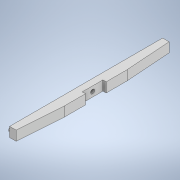
# Autodesk Inventor part: atx_mount
Saved by Autodesk Inventor 2022 (Build 260153000, 153)
## iProperties
Created: 2021-12-15
Part Number: atx_mount
Material: Generisch
Document SubType Name: Modeling
Designer: Niclas
Density: 1 g/cm^3
Appearance: Vorgabe
Author: Niclas
Autodesk Inventor part; units mm, degrees
ref_plane "YZ Plane" through (0, 0, 0) normal (1, 0, 0) x (0, 1, 0)
ref_plane "XZ Plane" through (0, 0, 0) normal (0, 1, 0) x (-1, 0, 0)
ref_plane "XY Plane" through (0, 0, 0) normal (0, 0, 1) x (1, 0, 0)
sketch "Skizze3" plane through (0, 0, 0) normal (0, 1, 0) x (-1, 0, 0)
  line L0 (15, 237) -> (0, 237)
  line L1 (0, 237) -> (0, 0)
  line L2 (0, 0) -> (15, 0)
  line L3 (15, 0) -> (15, 237)
  line L4 (5, 134.5) -> (0, 134.5)
  line L5 (0, 134.5) -> (0, 102.5)
  line L6 (0, 102.5) -> (5, 102.5)
  line L7 (5, 102.5) -> (5, 134.5)
  point P0 (0, 134.5)
  dimension "d17" = 237
  dimension "d18" = 15
  dimension "d19" = 5
  dimension "d20" = 32
  dimension "d69" = 102.5
  constraints: 16 end point, 4 parallel, 2 horizontal, 2 perpendicular, 1 coincident, 1 point on line
  measures "d17" distance of L2.end L0.start
  measures "d18" distance of L1.end L2.end
  measures "d19" distance of L5.end L6.end
  measures "d20" distance between parallel lines of L6 L4
  measures "d69" distance between parallel lines of L2 L6
extrude "Extrusion4" add sketch "Skizze3" along normal blind 15 contours L3 L2 L1 L6 L7 L4 L0
sketch "Skizze6" plane through (0, 0, 0) normal (0, -1, 0) x (1, 0, 0)
  line L0 (0, 70) -> (-5, 0)
  line L1 (0, 0) -> (-15, 0) projected
  line L2 (0, 102.5) -> (0, 0) projected
  line L3 (-5, 237) -> (0, 167)
  line L4 (-15, 237) -> (0, 237) projected
  line L5 (0, 237) -> (0, 134.5) projected
  point P0 (0, 167)
  dimension "d48" = 0
  dimension "d49" = 10
  dimension "d50" = 0
  dimension "d51" = 70
  dimension "d52" = 0
  dimension "d53" = 10
  dimension "d54" = 70
  dimension "d55" = 0
  constraints: 4 end point
  measures "d48" distance from line of L1 L0.end
  measures "d49" distance of L1.end L0.end
  measures "d50" distance from line of L2 L0.start
  measures "d51" distance of L0.start L1.start
  measures "d52" distance from line of L4 L3.start
  measures "d53" distance of L4.start L3.start
  measures "d54" distance of L4.end L3.end
  measures "d55" distance from line of L3.end L5
extrude "Extrusion9" cut sketch "Skizze6" against normal blind 20
sketch "Skizze9" plane through (-15, 0, 0) normal (-1, 0, 0) x (0, 0, 1)
  circle A0 centre (118.5, 7.5) radius 3.1
  line L0 (0, 0) -> (0, 15) projected
  line L1 (0, 15) -> (237, 15) projected
  dimension "d70" = 6.2
  dimension "d71" = 118.5
  dimension "d72" = 7.5
  constraints: 1 centre point
  measures "d70" diameter of A0
  measures "d71" distance from line of L0 A0.centre
  measures "d72" distance from line of L1 A0.centre
extrude "Extrusion12" cut sketch "Skizze9" against normal blind 10
sketch "Skizze10" plane through (-15, 0, 0) normal (-1, 0, 0) x (0, 0, 1)
  circle A0 centre (4.8, 7.5) radius 2.3
  line L0 (0, 15) -> (237, 15) projected
  circle A1 centre (159.74, 7.5) radius 2.3
  circle A2 centre (232.13, 7.5) radius 2.3
  circle A3 centre (27.66, 7.5) radius 2.3
  line L1 (0, 0) -> (0, 15) projected
  dimension "d80" = 4.6
  dimension "d84" = 7.5
  dimension "d85" = 4.6
  dimension "d86" = 4.6
  dimension "d87" = 4.6
  dimension "d88" = 227.33
  dimension "d89" = 4.8
  dimension "d90" = 7.5
  dimension "d91" = 22.86
  dimension "d92" = 7.5
  dimension "d93" = 154.94
  dimension "d94" = 7.5
  constraints: 4 centre point
  measures "d80" diameter of A0
  measures "d84" distance from line of L0 A0.centre
  measures "d85" diameter of A3
  measures "d86" diameter of A1
  measures "d87" diameter of A2
  measures "d88" distance of A2.centre A0.centre
  measures "d89" distance from line of L1 A0.centre
  measures "d90" distance from line of L0 A2.centre
  measures "d91" distance of A0.centre A3.centre
  measures "d92" distance from line of L0 A3.centre
  measures "d93" distance of A0.centre A1.centre
  measures "d94" distance from line of L0 A1.centre
sketch "Skizze11" plane through (-15, 0, 0) normal (-1, 0, 0) x (0, 0, 1)
  circle A0 centre (118.5, 7.5) radius 3.1 projected
  circle A1 centre (118.5, 7.5) radius 6
  point P0 (0, 0)
  dimension "d81" = 12
  constraints: 1 centre point, 1 coincident
  measures "d81" diameter of A1
extrude "Extrusion15" cut sketch "Skizze11" against normal blind 5
extrude "Extrusion16" cut sketch "Skizze10" against normal blind 8
sketch "Skizze12" plane through (-15, 0, 0) normal (-1, 0, 0) x (0, 0, 1)
  circle A0 centre (159.74, 7.5) radius 2.3 projected
  circle A1 centre (232.13, 7.5) radius 2.3 projected
  circle A2 centre (27.66, 7.5) radius 2.3 projected
  circle A3 centre (4.8, 7.5) radius 2.3 projected
  circle A4 centre (232.13, 7.5) radius 2.3 projected
  circle A5 centre (232.13, 7.5) radius 3.5
  circle A6 centre (159.74, 7.5) radius 2.3 projected
  circle A7 centre (159.74, 7.5) radius 3.5
  circle A8 centre (27.66, 7.5) radius 3.5
  circle A9 centre (4.8, 7.5) radius 3.5
  point P0 (0, 0)
  dimension "d97" = 7
  dimension "d98" = 7
  dimension "d99" = 7
  dimension "d100" = 7
  constraints: 4 centre point, 4 coincident
  measures "d97" diameter of A5
  measures "d98" diameter of A7
  measures "d99" diameter of A8
  measures "d100" diameter of A9
extrude "Extrusion17" add sketch "Skizze12" along normal blind 3
chamfer "Fase3" distance 1.5 angle 45 4 edges at (-15, 7.5, 228.63) (-15, 7.5, 156.24) (-15, 7.5, 24.16) (-15, 7.5, 1.3)
